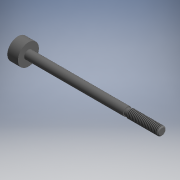
# Autodesk Inventor part: 10_11-CJ2B10-15Z_ROD
Saved by Autodesk Inventor 2017.3 (Build 213256000, 256)
## iProperties
Part Number: 10_11-CJ2B10-15Z_ROD
Material: Generic
Catalog Web Link: www.cadenas.de
Description: 10/11-CJ2-Z ROD-Air Cylinder/Standard: Double Acting Single Rod/Clean Series
Vendor: SMC
Document SubType Name: Modeling
Designer: partserver
Manufacturer: SMC
Mass: 1.18357 g
Surface Area: 11.1345 cm^2
Volume: 1.18357 cm^3
Density: 1 g/cm^3
Appearance: PSOLRGB-128-128-128
Category: PARTsolutions
Company: SMC
Title: 10_11-CJ2B10-15Z_ROD
Author: Cadenas PARTsolutions
Comments: Air Cylinder/Standard: Double Acting Single Rod/Clean Series
PSOL_IDENT_0: {$CADENAS_DATA\23d-libs\smc_jp\actuator\standard_air_cylinder\cj2\10_cj2_z\parts\10_cj2_z_rod.prj},2
PSOL_IDENT_1: 02 {VTYP=3D},{NB=10_11-CJ2B10-15Z_ROD},{LINA=10_11-CJ2B10-15Z_ROD},{NN=10/11-CJ2-Z ROD},{DATE=29.10.
PSOL_IDENT_2: 2021 06:22:38},{GEOMDATE=05.06.2020 09:38:22},{VERSION=},{LINEID=370},{WBVAR=STROKE},{WBNUMERIC=STRO
PSOL_IDENT_3: KE}  {NB=10_11-CJ2B10-15Z_ROD},{LINA=10_11-CJ2B10-15Z_ROD},{KT=DUMMY},{ORDER=10_11-CJ2B10-15Z},{BORE=
PSOL_IDENT_4: 10},{MOUNT=(B) Basic},{MOUNTX=B},{STROKE=15},{A=15},{D=4},{H=28},{MM=M4x0.7},{MM1=4},{MM2=0.7},{NA=2
PSOL_IDENT_5: 0.5},{NA1=20.5},{S=54},{S1=54.000},{NB1=9.500},{SMAX=150.000}
NB: 10_11-CJ2B10-15Z_ROD
NN: 10/11-CJ2-Z ROD
NT: Air Cylinder/Standard: Double Acting Single Rod/Clean Series
NBSYN: $ORDER._ROD
LINA: 10_11-CJ2B10-15Z_ROD
CATALOG: SMC (JP
BORE: 10
MOUNT: (B) Basic
STROKE: 15
A: 15
D: 4
H: 28
MM: M4x0.7
MM1: 4
MM2: 0.7
NA1: 20.5
S1: 54
NB1: 9.5
SMAX: 150
SUPPLIER: SMC
ARTICLENO: 10_11-CJ2B10-15Z_ROD
BOMINFO: 10_11-CJ2B10-15Z_ROD
CREATOR: CADENAS GmbH
Autodesk Inventor part; units mm, degrees
sketch "Sketch_2" plane through (0, 0, 0) normal (0, 0, 1) x (1, 0, 0)
  line L0 (68.5, 0) -> (0, 0)
  line L1 (0, 0) -> (0, 1.5705)
  line L2 (0, 1.5705) -> (0.4295, 2)
  line L3 (0.4295, 2) -> (15, 2)
  line L4 (15, 2) -> (15, 1.65)
  line L5 (15, 1.65) -> (16.5, 1.65)
  line L6 (16.5, 1.65) -> (16.5, 2)
  line L7 (16.5, 2) -> (63.5, 2)
  line L8 (63.5, 2) -> (63.5, 5)
  line L9 (63.5, 5) -> (68.5, 5)
  line L10 (68.5, 5) -> (68.5, 0)
  line L11 (68.5, 0) -> (0, 0)
  constraints: 24 end point
revolve "Revolution1" add sketch "Sketch_2" angle 360 about axis through (68.5, 0, 0) along (1, 0, 0)
thread "Thread1" size "M4x0.7" class "6g" standard "ISO Metric profile" full length
ref_plane "ROD_BA_XY" through (8, 0, 0) normal (-1, 0, 0) x (0, 0, -1)
ref_plane "ROD_BA_YZ" through (8, 0, 0) normal (0, 0, -1) x (0, -1, 0)
ref_plane "ROD_BA_ZX" through (8, 0, 0) normal (0, -1, 0) x (-1, 0, 0)
ref_plane "ROD_BODY_XY" through (28, 0, 0) normal (-1, 0, 0) x (0, 0, -1)
ref_plane "ROD_BODY_YZ" through (28, 0, 0) normal (0, 0, -1) x (0, -1, 0)
ref_plane "ROD_BODY_ZX" through (28, 0, 0) normal (0, -1, 0) x (-1, 0, 0)
ref_plane "rodnt1_XY" through (7.5, 0, 0) normal (1, 0, 0) x (0, 0, -1)
ref_plane "rodnt1_YZ" through (7.5, 0, 0) normal (0, 0, -1) x (0, 1, 0)
ref_plane "rodnt1_ZX" through (7.5, 0, 0) normal (0, 1, 0) x (1, 0, 0)
body "Solid1"
